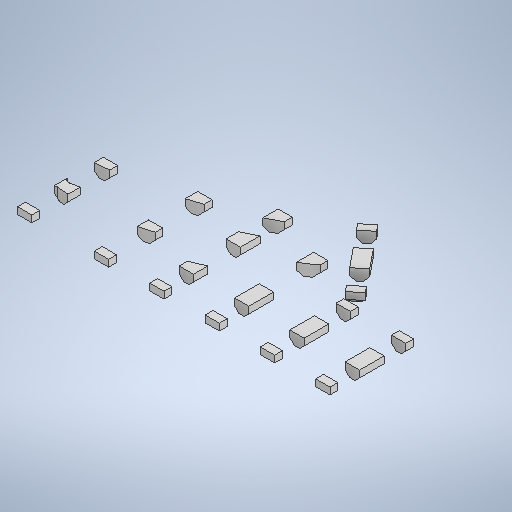
# Autodesk Inventor part: RR_SingleTurnout_Pillow
Saved by Autodesk Inventor 2025.1 (Build 291241000, 241)
## iProperties
Created: 2025-03-08
Part Number: RR_SingleTurnout_Pillow
Material: 一般
Document SubType Name: Modeling
Designer: kumagai
Density: 1 g/cm^3
Appearance: 既定
Author: kumagai
Autodesk Inventor part; units mm, degrees
ref_plane "YZ Plane" through (0, 0, 0) normal (1, 0, 0) x (0, 1, 0)
ref_plane "XZ Plane" through (0, 0, 0) normal (0, 1, 0) x (-1, 0, 0)
ref_plane "XY Plane" through (0, 0, 0) normal (0, 0, 1) x (1, 0, 0)
derived "RR_SingleTurnout.ipt"
sketch "MainSketch" plane through (0, 0, 0) normal (0, 1, 0) x (-1, 0, 0)
  line L0 (0, -306.513602) -> (0, 56.948342)
  line L1 (-275.368476, 0) -> (77.210854, 0)
  line L2 (14.635918, -29) -> (-5, -29)
  line L3 (-5, -49.510649) -> (-5, -5.641597)
  line L4 (-5, -48) -> (0, -48)
  line L5 (-5, -10) -> (0, -10)
  line L6 (-5, -38.3) -> (0, -38.3)
  line L7 (-5, -19.7) -> (0, -19.7)
  line L8 (-5, -46) -> (0, -46)
  line L9 (-5, -35.9) -> (0, -35.9)
  line L10 (-5, -22.1) -> (0, -22.1)
  line L11 (-5, -12) -> (0, -12)
  line L12 (-10, -10) -> (-225, -10)
  line L13 (-10, -10) -> (-10, -48)
  line L14 (-225, -48) -> (-225, -10)
  line L15 (-10, -12) -> (-225, -12)
  line L16 (-93.096355, -19.7) -> (-225, -19.7)
  arc A0 (-10, -48) -> (-148.592929, -105.407071) centre (-10, -244) ccw
  arc A1 (-10, -46) -> (-150.007143, -103.992857) centre (-10, -244) ccw
  line L17 (-143.221471, -110.778529) -> (-189.510214, -64.489786)
  line L18 (-210, -35.9) -> (-210, -22.1)
  line L19 (-146.159556, -86.627241) -> (-155.94149, -76.845307)
  arc A2 (-133.884663, -47.845494) -> (-174.048773, -79.951227) centre (-10, -244) ccw
  arc A3 (-139.222917, -48.916844) -> (-175.462987, -78.537013) centre (-10, -244) ccw
  line L20 (-139.499035, -48) -> (-225, -48)
  line L21 (-134.418648, -46) -> (-225, -46)
  arc A4 (-118.910301, -50.665688) -> (-166.906995, -87.093005) centre (-10, -244) ccw
  arc A5 (-120.08824, -48.574645) -> (-168.604051, -85.395949) centre (-10, -244) ccw
  line L22 (-88.399738, -46) -> (-110.27208, -46)
  arc A6 (-91.807872, -26.90216) -> (-113.191266, -36.212698) centre (-10, -244) ccw
  line L23 (-122.087064, -35.9) -> (-225, -35.9)
  line L24 (-122.087064, -38.3) -> (-225, -38.3)
  arc A7 (-133.884663, -47.845494) -> (-134.418648, -46) centre (-134.418648, -47) ccw
  arc A8 (-139.222917, -48.916844) -> (-139.499035, -48) centre (-139.499035, -48.5) ccw
  arc A9 (-110.27208, -48.4) -> (-118.910301, -50.665688) centre (-110.27208, -66) ccw
  arc A10 (-110.27208, -46) -> (-120.08824, -48.574645) centre (-110.27208, -66) ccw
  arc A11 (-122.087064, -38.3) -> (-113.191266, -36.212698) centre (-122.087064, -18.3) ccw
  arc A12 (-122.087064, -35.9) -> (-114.258761, -34.063175) centre (-122.087064, -18.3) ccw
  arc A13 (-84.356493, -34.928907) -> (-84.188948, -35.9) centre (-84.188948, -35.4) ccw
  arc A14 (-94.86504, -36.374339) -> (-94.486685, -38.3) centre (-94.486685, -37.3) ccw
  arc A15 (-103.925858, -28.586599) -> (-108.30509, -30.549516) centre (-10, -244) ccw
  arc A16 (-92.200549, -21.144444) -> (-91.472655, -25.240528) centre (-89.065226, -22.7) ccw
  arc A17 (-95.293597, -25.669145) -> (-114.258761, -34.063175) centre (-10, -244) ccw
  line L25 (-95.953622, -22.1) -> (-225, -22.1)
  arc A18 (-94.955304, -23.042029) -> (-94.702079, -24.442381) centre (-89.065226, -22.7) ccw
  arc A19 (-91.807872, -26.90216) -> (-91.472655, -25.240528) centre (-92.160492, -25.966394) ccw
  arc A20 (-92.200549, -21.144444) -> (-93.096355, -19.7) centre (-93.096355, -20.7) ccw
  arc A21 (-95.293597, -25.669145) -> (-94.702079, -24.442381) centre (-95.657478, -24.737699) ccw
  arc A22 (-94.955304, -23.042029) -> (-95.953622, -22.1) centre (-95.953622, -23.1) ccw
  circle A23 centre (-89.065226, -22.7) radius 2.5
  arc A24 (-96.002889, -53.844292) -> (-104.887042, -58.117943) centre (-10, -244) ccw
  arc A25 (-90.258687, -49.342029) -> (-89.9638, -50.871855) centre (-84.368609, -49) ccw
  arc A26 (-87.503931, -47.444444) -> (-86.718807, -51.593563) centre (-84.368609, -49) ccw
  arc A27 (-90.525183, -52.111217) -> (-157.148921, -96.851079) centre (-10, -244) ccw
  line L26 (-91.257005, -48.4) -> (-110.27208, -48.4)
  arc A28 (-87.015883, -53.261845) -> (-155.451865, -98.548135) centre (-10, -244) ccw
  arc A29 (-87.015883, -53.261845) -> (-86.718807, -51.593563) centre (-87.390292, -52.334581) ccw
  arc A30 (-87.503931, -47.444444) -> (-88.399738, -46) centre (-88.399738, -47) ccw
  arc A31 (-90.525183, -52.111217) -> (-89.9638, -50.871855) centre (-90.912137, -51.189118) ccw
  arc A32 (-90.258687, -49.342029) -> (-91.257005, -48.4) centre (-91.257005, -49.4) ccw
  circle A33 centre (-84.368609, -49) radius 2.5
  line L27 (-43.456838, -12) -> (-26.685323, -12)
  arc A34 (-26.663775, -12.599225) -> (-88.055883, -25.525106) centre (-10, -244) ccw
  arc A35 (-89.065226, -19.7) -> (-88.055883, -25.525106) centre (-89.065226, -22.7) ccw
  arc A36 (-26.663775, -12.599225) -> (-26.685323, -12) centre (-26.685323, -12.3) ccw
  arc A37 (-43.456838, -12) -> (-76.688171, -19.286743) centre (-10, -244) ccw
  line L28 (-89.065226, -19.7) -> (-79.533229, -19.7)
  arc A38 (-79.533229, -19.7) -> (-76.688171, -19.286743) centre (-79.533229, -9.7) ccw
  circle A39 centre (-84.368609, -49) radius 3
  line L29 (-84.957689, -46.058404) -> (-27.151089, -34.482133)
  arc A40 (-27.010586, -35.064983) -> (-41.702277, -39.843786) centre (26.842379, -225.600697) ccw
  arc A41 (-27.010586, -35.064983) -> (-27.151089, -34.482133) centre (-27.092181, -34.776293) ccw
  arc A42 (-74.693989, -46.707276) -> (-82.769984, -51.538582) centre (26.842379, -225.600697) ccw
  line L30 (-73.207719, -46.153023) -> (-41.702277, -39.843786)
  arc A43 (-73.207719, -46.153023) -> (-74.693989, -46.707276) centre (-72.225919, -51.055682) ccw
  arc A44 (-48.487832, -13.997985) -> (-81.659642, -22.083043) centre (-10, -244) ccw
  arc A45 (-27.985942, -39.087834) -> (-44.461342, -41.207234) centre (-10, -244) ccw
  line L31 (-33.091622, -19.7) -> (-48.022721, -19.7)
  line L32 (-25.839787, -35.987884) -> (-26.168788, -34.398641)
  line L33 (-26.759766, -34.010381) -> (-46.4779, -38.09237)
  line L34 (-46.964425, -35.742201) -> (-27.24629, -31.660213)
  line L35 (-23.818619, -33.912116) -> (-23.489619, -35.501359)
  line L36 (-10, -38.3) -> (-23, -38.3)
  line L37 (-48.505087, -38.3) -> (-94.486685, -38.3)
  line L38 (-10, -35.9) -> (-23, -35.9)
  line L39 (-48.505087, -35.9) -> (-84.188948, -35.9)
  arc A46 (-25.839787, -35.987884) -> (-23, -38.3) centre (-23, -35.4) ccw
  arc A47 (-23.489619, -35.501359) -> (-23, -35.9) centre (-23, -35.4) ccw
  arc A48 (-23.818619, -33.912116) -> (-27.24629, -31.660213) centre (-26.658406, -34.5) ccw
  arc A49 (-26.168788, -34.398641) -> (-26.759766, -34.010381) centre (-26.658406, -34.5) ccw
  arc A50 (-48.505087, -38.3) -> (-46.4779, -38.09237) centre (-48.505087, -28.3) ccw
  arc A51 (-48.505087, -35.9) -> (-46.964425, -35.742201) centre (-48.505087, -28.3) ccw
  arc A52 (-10, -22.1) -> (-22.0271, -22.426177) centre (-10, -244) ccw
  arc A53 (-46.74201, -25.162995) -> (-84.356493, -34.928907) centre (-10, -244) ccw
  arc A54 (-10, -19.7) -> (-22.157182, -20.029705) centre (-10, -244) ccw
  arc A55 (-47.1394, -22.796123) -> (-94.86504, -36.374339) centre (-10, -244) ccw
  arc A56 (-25.454973, -23.996969) -> (-45.236808, -22.661135) centre (-50.962587, -254.590467) ccw
  line L40 (-24.9, -22.925442) -> (-24.9, -23.5)
  arc A57 (-25.454973, -23.996969) -> (-24.9, -23.5) centre (-25.4, -23.5) ccw
  arc A58 (-22.157182, -20.029705) -> (-24.9, -22.925442) centre (-22, -22.925442) ccw
  arc A59 (-45.236808, -22.661135) -> (-47.1394, -22.796123) centre (-45.483608, -32.658089) ccw
  arc A60 (-25.718845, -26.382419) -> (-45.29604, -25.060404) centre (-50.962587, -254.590467) ccw
  arc A61 (-22.0271, -22.426177) -> (-22.5, -22.925442) centre (-22, -22.925442) ccw
  line L41 (-22.5, -22.925442) -> (-22.5, -23.5)
  arc A62 (-25.718845, -26.382419) -> (-22.5, -23.5) centre (-25.4, -23.5) ccw
  arc A63 (-45.29604, -25.060404) -> (-46.74201, -25.162995) centre (-45.483608, -32.658089) ccw
  line L42 (-51.7, -52.487311) -> (-51.7, -10)
  line L43 (-44.3, -51.024587) -> (-44.3, -10)
  line L44 (-48, 3.351653) -> (-48, 5.025207)
  line L45 (-59, -53) -> (-37, -53)
  line L46 (-59, -8.2) -> (-37, -8.2)
  line L47 (-37, -8.2) -> (-37, 0.8)
  line L48 (-40, 3.8) -> (-42, 3.8)
  line L49 (-42, 3.8) -> (-40, -7.7)
  line L50 (-40, -7.7) -> (-56, -7.7)
  line L51 (-56, -7.7) -> (-54, 3.8)
  line L52 (-54, 3.8) -> (-56, 3.8)
  line L53 (-59, 0.8) -> (-59, -8.2)
  line L54 (-37, -8.2) -> (-37, -10)
  line L55 (-59, -8.2) -> (-59, -10)
  arc A64 (-37, 0.8) -> (-40, 3.8) centre (-40, 0.8) ccw
  arc A65 (-56, 3.8) -> (-59, 0.8) centre (-56, 0.8) ccw
  line L56 (-44.3, -10) -> (-44.3, -7.7)
  line L57 (-51.7, -10) -> (-51.7, -7.7)
  line L58 (-48, -62.11824) -> (-48, -64.382845)
  line L59 (-37, -53) -> (-37, -62)
  line L60 (-40, -65) -> (-42, -65)
  line L61 (-42, -65) -> (-40, -53.5)
  line L62 (-40, -53.5) -> (-56, -53.5)
  line L63 (-56, -53.5) -> (-54, -65)
  line L64 (-54, -65) -> (-56, -65)
  line L65 (-59, -62) -> (-59, -53)
  arc A66 (-40, -65) -> (-37, -62) centre (-40, -62) ccw
  arc A67 (-59, -62) -> (-56, -65) centre (-56, -62) ccw
  line L66 (-37, -53) -> (-37, -49.868601)
  line L67 (-44.3, -51.024587) -> (-44.3, -53.5)
  line L68 (-51.7, -52.487311) -> (-51.7, -53.5)
  arc A68 (-34.373057, -49.521327) -> (-37, -52.498042) centre (-34, -52.498042) ccw
  arc A69 (-59, -58.137147) -> (-62.80829, -55.248087) centre (-62, -58.137147) ccw
  arc A70 (-37, -7) -> (-34, -10) centre (-34, -7) ccw
  arc A71 (-62, -10) -> (-59, -7) centre (-62, -7) ccw
  point P0 (0, 0)
  point P1 (-90.868002, -19.7)
  point P2 (-94.934638, -22.1)
  point P3 (-90.238021, -48.4)
  point P4 (-86.171385, -46)
  point P5 (-162.027958, -91.972042)
  point P6 (-225, -29)
  point P7 (-10, -29)
  point P8 (-48.583504, -39.997985)
  point P9 (-48, 2.002015)
  point P10 (-48, -55.997985)
  point P11 (-37, 3.8)
  point P12 (-59, 3.8)
  point P13 (-37, -65)
  point P14 (-59, -65)
sketch "PillowSketch" plane through (0, 0, 0) normal (0, 1, 0) x (-1, 0, 0)
  arc A0 (-10, -48) -> (-148.592929, -105.407071) centre (-10, -244) ccw
  arc A1 (-139.222917, -48.916844) -> (-175.462987, -78.537013) centre (-10, -244) ccw
  line L0 (-139.499035, -48) -> (-225, -48)
  line L1 (-10, -10) -> (-225, -10)
  line L2 (-143.221471, -110.778529) -> (-189.510214, -64.489786)
  line L3 (-225, -48) -> (-225, -10)
  line L4 (-10, -10) -> (-10, -48)
  line L5 (-122.087064, -35.9) -> (-225, -35.9)
  line L6 (-95.953622, -22.1) -> (-225, -22.1)
  arc A2 (-95.293597, -25.669145) -> (-114.258761, -34.063175) centre (-10, -244) ccw
  arc A3 (-46.74201, -25.162995) -> (-84.356493, -34.928907) centre (-10, -244) ccw
  line L7 (-48.505087, -35.9) -> (-84.188948, -35.9)
  line L8 (-46.964425, -35.742201) -> (-27.24629, -31.660213)
  arc A4 (-25.718845, -26.382419) -> (-45.29604, -25.060404) centre (-50.962587, -254.590467) ccw
  line L9 (-40, -1.453398) -> (-40, 7.794531)
  line L10 (-71, -1.742094) -> (-71, 3.022862)
  line L11 (-102, -0.652961) -> (-102, 5.473411)
  line L12 (-133, -1.049652) -> (-133, 3.46415)
  line L13 (-164, -2.883385) -> (-164, 3.46415)
  line L14 (-195, -2.812134) -> (-195, 3.533956)
  line L15 (-121.433249, -106.391398) -> (-109.724259, -120.850796)
  line L16 (-101.818669, -89.666692) -> (-92.425581, -105.455055)
  line L17 (-79.395346, -76.464815) -> (-71.186837, -96.281907)
  line L18 (-67, -5.6) -> (-75, -5.6)
  line L19 (-75, -63.491915) -> (-67, -63.491915)
  line L20 (-98, -5.6) -> (-106, -5.6)
  line L21 (-106, -77.519925) -> (-98, -77.519925)
  line L22 (-156.899881, -56.237692) -> (-163.117048, -61.272255)
  line L23 (-133.660682, -97.647839) -> (-127.443514, -92.613276)
  line L24 (-129, -5.6) -> (-137, -5.6)
  line L25 (-137, -66.436789) -> (-129, -66.436789)
  arc A5 (-90.525183, -52.111217) -> (-157.148921, -96.851079) centre (-10, -244) ccw
  arc A6 (-118.910301, -50.665688) -> (-166.906995, -87.093005) centre (-10, -244) ccw
  line L26 (-160, -5.6) -> (-168, -5.6)
  line L27 (-168, -52.4) -> (-160, -52.4)
  line L28 (-191, -5.6) -> (-199, -5.6)
  line L29 (-199, -52.4) -> (-191, -52.4)
  line L30 (-160, -52.4) -> (-160, -48)
  line L31 (-168, -48) -> (-168, -52.4)
  line L32 (-191, -52.4) -> (-191, -48)
  line L33 (-199, -48) -> (-199, -52.4)
  line L34 (-199, -5.6) -> (-199, -10)
  line L35 (-199, -22.1) -> (-199, -35.9)
  line L36 (-191, -35.9) -> (-191, -22.1)
  line L37 (-191, -10) -> (-191, -5.6)
  line L38 (-168, -5.6) -> (-168, -10)
  line L39 (-168, -22.1) -> (-168, -35.9)
  line L40 (-160, -35.9) -> (-160, -22.1)
  line L41 (-160, -10) -> (-160, -5.6)
  line L42 (-137, -62.036789) -> (-137, -66.436789)
  line L43 (-129, -66.436789) -> (-129, -56.707154)
  line L44 (-129, -35.9) -> (-129, -22.1)
  line L45 (-129, -10) -> (-129, -5.6)
  line L46 (-137, -5.6) -> (-137, -10)
  line L47 (-137, -22.1) -> (-137, -35.9)
  line L48 (-91.257005, -48.4) -> (-110.27208, -48.4)
  line L49 (-98, -10) -> (-98, -5.6)
  line L50 (-106, -5.6) -> (-106, -10)
  line L51 (-98, -26.745863) -> (-98, -22.1)
  line L52 (-106, -22.1) -> (-106, -30.160434)
  line L53 (-98, -77.519925) -> (-98, -68.865766)
  line L54 (-98, -55.422138) -> (-98, -48.4)
  line L55 (-106, -48.4) -> (-106, -59.366282)
  line L56 (-106, -73.119925) -> (-106, -77.519925)
  line L57 (-67, -63.491915) -> (-67, -56.471336)
  line L58 (-75, -59.091915) -> (-75, -63.491915)
  line L59 (-75, -5.6) -> (-75, -10)
  line L60 (-75, -31.833532) -> (-75, -35.9)
  line L61 (-67, -35.9) -> (-67, -29.545786)
  line L62 (-67, -10) -> (-67, -5.6)
  line L63 (-28, -2.749625) -> (-28, 7.336921)
  line L64 (-24, -5.6) -> (-32, -5.6)
  line L65 (-32, -53.638608) -> (-24, -53.638608)
  arc A7 (-23.818619, -33.912116) -> (-27.24629, -31.660213) centre (-26.658406, -34.5) ccw
  arc A8 (-25.718845, -26.382419) -> (-22.5, -23.5) centre (-25.4, -23.5) ccw
  line L66 (-24, -53.638608) -> (-24, -48.500639)
  line L67 (-32, -49.238608) -> (-32, -53.638608)
  line L68 (-24, -33.341175) -> (-24, -26.039685)
  line L69 (-24, -10) -> (-24, -5.6)
  line L70 (-32, -5.6) -> (-32, -10)
  line L71 (-32, -25.774864) -> (-32, -32.644311)
  line L72 (-136.429691, -94.228397) -> (-133.660682, -97.647839)
  line L73 (-127.443514, -92.613276) -> (-130.212524, -89.193834)
  line L74 (-163.117048, -61.272255) -> (-160.348039, -64.691698)
  line L75 (-152.732088, -74.096613) -> (-144.045962, -84.823086)
  line L76 (-137.828794, -79.788522) -> (-146.514921, -69.06205)
  line L77 (-154.130871, -59.657134) -> (-156.899881, -56.237692)
  point P0 (0, 0)
  dimension "d1" = 30
  dimension "d2" = 31
  dimension "d3" = 31
  dimension "d4" = 31
  dimension "d5" = 31
  dimension "d6" = 31
  dimension "d7" = 30
  dimension "d8" = 6
  dimension "d9" = 8.25
  dimension "d10" = 8.25
  dimension "d11" = 8
  dimension "d12" = 4.4
  dimension "d13" = 4.4
  dimension "d14" = 8
  dimension "d16" = 8
  dimension "d17" = 4.4
  dimension "d18" = 8
  dimension "d19" = 4.4
  dimension "d20" = 8
  dimension "d21" = 4.4
  dimension "d22" = 18
  dimension "d24" = 8
  dimension "d25" = 4.4
  dimension "d27" = 8
  dimension "d28" = 4.4
  dimension "d29" = 4.4
  constraints: 136 end point, 36 collinear, 19 point on line, 17 point on circle, 6 perpendicular, 6 vertical, 4 horizontal, 3 parallel, 38 other
  measures "d1" distance between parallel lines of L3 L14
  measures "d2" distance between parallel lines of L13 L14
  measures "d3" distance between parallel lines of L12 L13
  measures "d4" distance between parallel lines of L11 L12
  measures "d5" distance between parallel lines of L11 L10
  measures "d6" distance between parallel lines of L9 L10
  measures "d7" distance between parallel lines of L4 L9
  measures "d8" angle of L15 L2
  measures "d9" angle of L16 L15
  measures "d10" angle of L17 L16
  measures "d11" distance between parallel lines of L34 L37
  measures "d13" distance between parallel lines of L29 L0
  measures "d14" distance between parallel lines of L38 L41
  measures "d16" distance between parallel lines of L46 L45
  measures "d17" distance of L42.start L25.start
  measures "d18" distance between parallel lines of L50 L49
  measures "d19" distance of L56.start L21.start
  measures "d20" distance between parallel lines of L59 L62
  measures "d21" distance of L58.start L19.start
  measures "d22" distance between parallel lines of L4 L63
  measures "d24" distance between parallel lines of L70 L69
  measures "d25" distance of L65.start L67.start
  measures "d27" distance between parallel lines of L73 L72
  measures "d28" distance of L72.start L23.start
  measures "d29" distance of L22.end L74.end
extrude "PillowBody" add sketch "PillowSketch" along normal blind 2.1 and the other way blind 4.2 contours L66 L65 L67 A0 | L57 L19 L58 A0 | L53 L21 L56 A0 | L73 L23 L72 A0 | A1 L74 L22 L77 | L30 L27 L31 L0 | L32 L29 L33 L0 | L1 L70 L64 L69 | L1 L59 L18 L62 | L1 L50 L20 L49 | L1 L46 L24 L45 | L1 L38 L26 L41 | L1 L34 L28 L37 | L75 A6 L76 A5 | L35 L6 L36 L5 | L39 L6 L40 L5 | L47 L6 L44 L5 | L51 A2 L52 L6 | L61 L7 L60 A3 | L71 A4 A8 L68 A7 L8 | L42 A6 L43 L25 | A5 L55 L48 L54
chamfer "PillowChamfer" distance 2.5 angle 45 58 edges at (24, -4.2, -7.8) (32, -4.2, -7.8) (28, -4.2, -5.6) (32, -4.2, -29.2096) (24, -4.2, -29.6904) (24, -4.2, -51.0696) (28, -4.2, -53.6386) (32, -4.2, -51.4386) (67, -4.2, -7.8) (75, -4.2, -7.8) (71, -4.2, -5.6) (67, -4.2, -32.7229) (75, -4.2, -33.8668) (75, -4.2, -61.2919) (67, -4.2, -59.9816) (71, -4.2, -63.4919) (102, -4.2, -77.5199) (106, -4.2, -75.3199) (98, -4.2, -73.1928) (98, -4.2, -51.9111) (106, -4.2, -53.8831) (106, -4.2, -26.1302) (106, -4.2, -7.8) (102, -4.2, -5.6) (98, -4.2, -7.8) (129, -4.2, -7.8) (137, -4.2, -7.8) (133, -4.2, -5.6) (129, -4.2, -29) (137, -4.2, -29) (129, -4.2, -61.572) (133, -4.2, -66.4368) (137, -4.2, -64.2368) (142.1719, -4.2, -74.4253) (148.389, -4.2, -79.4598) (135.0452, -4.2, -95.9381) (128.828, -4.2, -90.9036) (130.5521, -4.2, -95.1306) (161.7325, -4.2, -62.982) (155.5154, -4.2, -57.9474) (160.0085, -4.2, -58.755) (164, -4.2, -52.4) (168, -4.2, -50.2) (160, -4.2, -50.2) (160, -4.2, -29) (168, -4.2, -29) (168, -4.2, -7.8) (164, -4.2, -5.6) (160, -4.2, -7.8) (191, -4.2, -7.8) (199, -4.2, -7.8) (195, -4.2, -5.6) (199, -4.2, -29) (191, -4.2, -29) (199, -4.2, -50.2) (195, -4.2, -52.4) (191, -4.2, -50.2) (98, -4.2, -24.4229)
